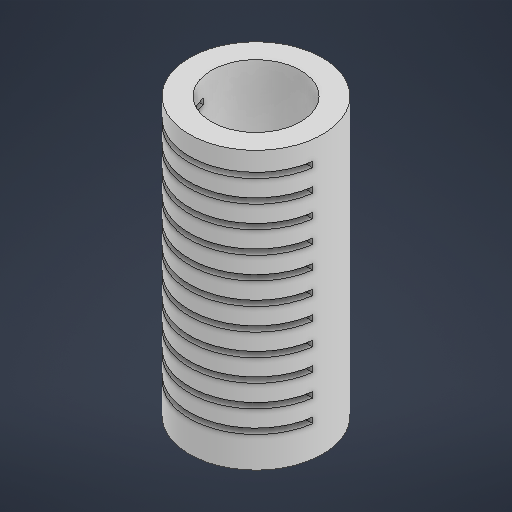
# Autodesk Inventor part: unión
Saved by Autodesk Inventor 2025.3 (Build 293356000, 356)
## iProperties
Created: 2025-11-05
Part Number: unión
Material: Genérico
Document SubType Name: Modeling
Designer: Jonathan Galarza
Density: 1 g/cm^3
Appearance: Valor por defecto
Author: Jonathan Galarza
Autodesk Inventor part; units mm, degrees
ref_plane "YZ Plane" through (0, 0, 0) normal (1, 0, 0) x (0, 1, 0)
ref_plane "XZ Plane" through (0, 0, 0) normal (0, 1, 0) x (-1, 0, 0)
ref_plane "XY Plane" through (0, 0, 0) normal (0, 0, 1) x (1, 0, 0)
sketch "Boceto1" plane through (0, 0, 0) normal (0, 1, 0) x (-1, 0, 0)
  circle A0 centre (0, 0) radius 4.025
  circle A1 centre (0, 0) radius 6
  dimension "d0" = 8.05
  dimension "d1" = 12
  constraints: 2 centre point, 2 coincident
  measures "d0" diameter of A0
  measures "d1" diameter of A1
extrude "Extrusión1" add sketch "Boceto1" along normal mid plane 25
sketch "Boceto2" plane through (0, 0, 0) normal (1, 0, 0) x (0, 1, 0)
  line L0 (10.7872, 7.1236) -> (10.2872, 7.1236)
  line L1 (10.2872, 7.1236) -> (10.2872, 0.8326)
  line L2 (10.2872, 0.8326) -> (10.7872, 0.8326)
  line L3 (10.7872, 0.8326) -> (10.7872, 7.1236)
  point P0 (0, 0)
  dimension "d4" = 0.5
  constraints: 8 end point, 2 parallel, 1 horizontal, 1 perpendicular
  measures "d4" distance of L2.end L1.end
extrude "Extrusión2" cut sketch "Boceto2" along normal mid plane 25
pattern_linear "Patrón rectangular1" count 11 spacing 2 along (0, -1, 0) of "Extrusión2"
